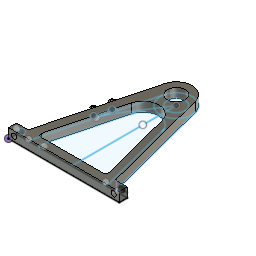
superstructure left v10 (Autodesk Fusion 360 design; units mm, degrees)
Autodesk Fusion 360 part; units mm, degrees
sketch "Sketch1" plane through (0, 0, 0) normal (0, 0, 1) x (1, 0, 0)
  line L0 (0, 0) -> (140, 0)
  line L1 (140, 0) -> (140, 10)
  line L2 (108.8274, 10) -> (31.1726, 10)
  line L3 (0, 10) -> (0, 0)
  line L4 (70, 10) -> (70, 142.1)
  circle A0 centre (70, 142.1) radius 11.2
  circle A1 centre (70, 142.1) radius 20
  line L5 (0, 10) -> (13.4534, 10)
  line L6 (140, 10) -> (126.5466, 10)
  line L7 (15.3891, 11.4969) -> (50.6432, 147.1312)
  line L8 (124.6109, 11.4969) -> (89.3568, 147.1312)
  line L9 (15, 10) -> (26, 10)
  line L10 (125, 10) -> (114, 10)
  line L11 (112.6988, 15.0062) -> (88.389, 108.5342)
  line L12 (27.3012, 15.0062) -> (51.611, 108.5342)
  arc A2 (27.3012, 15.0062) -> (31.1726, 10) centre (31.1726, 14) ccw
  arc A3 (108.8274, 10) -> (112.6988, 15.0062) centre (108.8274, 14) ccw
  arc A4 (13.4534, 10) -> (15.3891, 11.4969) centre (13.4534, 12) ccw
  arc A5 (124.6109, 11.4969) -> (126.5466, 10) centre (126.5466, 12) ccw
  line L13 (51.611, 108.5342) -> (50.6432, 104.8105)
  line L14 (88.389, 108.5342) -> (89.3568, 104.8105)
  arc A6 (89.3568, 104.8105) -> (50.6432, 104.8105) centre (70, 99.7793) ccw
  line L15 (70, 142.1) -> (35.085, 87.2735)
  line L16 (35.085, 87.2735) -> (37.4748, 96.468)
  line L17 (35.085, 87.2735) -> (32.6951, 78.0791)
  line L18 (37.4748, 96.468) -> (33.6034, 97.4743)
  circle A7 centre (33.6034, 97.4743) radius 2
  circle A8 centre (33.6034, 97.4743) radius 3.5
  line L19 (33.6034, 97.4743) -> (33.5258, 97.1755)
  line L20 (33.5258, 97.1755) -> (28.7461, 78.7865)
  circle A9 centre (28.7461, 78.7865) radius 2
  circle A10 centre (28.7461, 78.7865) radius 3.5
  line L21 (28.7461, 78.7865) -> (27.8656, 75.399)
  line L22 (29.6265, 82.1739) -> (33.4979, 81.1677)
  line L23 (27.8656, 75.399) -> (31.737, 74.3928)
  line L24 (33.6034, 97.4743) -> (34.4839, 100.8617)
  line L25 (34.4839, 100.8617) -> (38.3553, 99.8555)
  line L26 (32.723, 94.0868) -> (36.5943, 93.0806)
  dimension "d3" = 140
  dimension "d4" = 10
  dimension "d5" = 132.1
  dimension "d6" = 22.4
  dimension "d7" = 40
  dimension "d9" = 15
  dimension "d10" = 15
  dimension "d11" = 11
  dimension "d12" = 11
  dimension "d22" = 4
  dimension "d23" = 4
  dimension "d24" = 2
  dimension "d25" = 2
  dimension "d30" = 20
  dimension "d37" = 65
  dimension "d38" = 9.5
  dimension "d39" = 9.5
  dimension "d40" = 4
  dimension "d41" = 4
  dimension "d42" = 7
  dimension "d43" = 19
  dimension "d44" = 4
  dimension "d45" = 7
  constraint horizontal L0
  constraint vertical L1
  constraint horizontal L2
  constraint vertical L3
  constraint coincident L0.start L3.end
  constraint perpendicular L2 L4
  constraint coincident L4.end A0.centre
  constraint concentric A0 A1
  constraint perpendicular L3 L5
  constraint perpendicular L1 L6
  constraint coincident A1 L7.end
  constraint tangent A1 L7
  constraint coincident A1 L8.end
  constraint tangent A1 L8
  constraint parallel L2 L9
  constraint parallel L2 L10
  constraint parallel L8 L11
  constraint parallel L7 L12
  constraint coincident L2 L4.start
  constraint coincident L9.end L12
  constraint coincident L3.start L2
  constraint tangent L12 A2
  constraint tangent L2 A2
  constraint coincident L10.end L11
  constraint coincident L1.end L2
  constraint tangent L11 A3
  constraint tangent L2 A3
  constraint coincident L9.start L7
  constraint coincident L9.start L5
  constraint tangent L7 A4
  constraint tangent L5 A4
  constraint coincident L10.start L8
  constraint coincident L10.start L6
  constraint tangent L8 A5
  constraint tangent L6 A5
  constraint parallel L12 L13
  constraint parallel L11 L14
  constraint tangent L13 A6
  constraint tangent L14 A6
  constraint coincident L7 L15.end
  constraint parallel L7 L16
  constraint parallel L7 L17
  constraint perpendicular L7 L18
  constraint coincident L18.end A7.centre
  constraint concentric A7 A8
  constraint perpendicular L18 L19
  constraint parallel L17 L20
  constraint coincident L20.end A9.centre
  constraint concentric A9 A10
  constraint coincident A10 L21.end
  constraint parallel L20 L21
  constraint coincident A10 L22.start
  constraint coincident L20 L22.start
  constraint coincident L7 L22.end
  constraint perpendicular L7 L22
  constraint coincident L7 L23.end
  constraint tangent A10 L23
  constraint coincident A8 L24.end
  constraint perpendicular L18 L24
  constraint coincident L7 L25.end
  constraint tangent A8 L25
  constraint coincident A8 L26.start
  constraint coincident L20 L26.start
  constraint coincident L16 L26.end
  constraint perpendicular L7 L26
  measures "d3" distance of L0.start L0.end
  measures "d4" distance of L0.start L3.start
  measures "d5" distance of L4.start L4.end
  measures "d6" diameter of A0
  measures "d7" diameter of A1
  measures "d9" distance of L3.start L9.start
  measures "d10" distance of L1.end L10.start
  measures "d11" distance of L9.start L9.end
  measures "d12" distance of L10.start L10.end
  measures "d22" radius of A2
  measures "d23" radius of A3
  measures "d24" radius of A4
  measures "d25" radius of A5
  measures "d30" radius of A6
  measures "d37" distance of L4.end L15.end
  measures "d38" distance of L15.end L16.end
  measures "d39" distance of L15.end L17.end
  measures "d40" distance of L16.end L18.end
  measures "d41" diameter of A7
  measures "d42" diameter of A8
  measures "d43" distance of L19.end L20.end
  measures "d44" diameter of A9
  measures "d45" diameter of A10
extrude "Extrude1" add sketch "Sketch1" along normal blind 12 contours L0 L1 L3 A1 L5 L6 L7 L8 A4 A5 L15 L17 | L4 A0 A1 L15 | A1 L7 L15 L16 | L4 A0 A1 L15
sketch "Sketch2" plane through (0, 10, 0) normal (0, 1, 0) x (-1, 0, 0)
  line L0 (-140, 0) -> (-126.5466, 0)
  line L1 (-126.5466, 12) -> (-140, 12)
  line L2 (-140, 12) -> (-140, 0)
  line L3 (-140, 6) -> (-133, 6)
  circle A0 centre (-133, 6) radius 3.25
  line L4 (-126.5466, 0) -> (-126.5466, 12)
  line L5 (0, 6) -> (-7, 6)
  circle A1 centre (-7, 6) radius 3.25
  dimension "d16" = 7
  dimension "d18" = 6.5
  dimension "d27" = 6.5
  constraint midpoint L2 L3.start
  constraint perpendicular L2 L3
  constraint coincident L3.end A0.centre
  constraint perpendicular L4 L5
  constraint coincident L5.end A1.centre
  measures "d16" distance of L3.start L3.end
  measures "d18" diameter of A0
  measures "d27" diameter of A1
extrude "Extrude2" cut sketch "Sketch2" against normal blind 10 contours A0
extrude "Extrude3" cut sketch "Sketch2" against normal blind 10 contours A1
extrude "Extrude4" add sketch "Sketch1" along normal blind 9 contours L7 L17 A10 L22 L23 | L20 A9 A10 L21 | L20 A9 A10 L21 | L7 L18 A8 L25 | L18 A7 A8 L20 | A7 A8 L20 L24 | L7 L16 L18 A8 L26 | L18 A7 A8 L24
equation "superstructure_width = 140 mm"
equation "superstructure_height = 132.1 mm"
equation "d3 = superstructure_width"
equation "d5 = superstructure_height"
equation "hole_5m = 6.5 mm"
equation "d18 = hole_5m"
equation "d27 = hole_5m"
equation "d38 = ( 19 / 2 ) * 1 mm"
equation "d39 = ( 19 / 2 ) * 1 mm"
